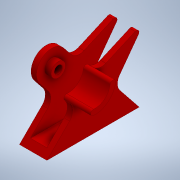
# Autodesk Inventor part: WeaponMountV1
Saved by Autodesk Inventor 2020 (Build 240168000, 168)
## iProperties
Created: 2024-02-06
Part Number: WeaponMountV1
Material: PETG
Document SubType Name: Modeling
Designer: smz3rm
Density: 1 g/cm^3
Appearance: Generic
Mass: 35.5696 g
Surface Area: 166.474 cm^2
Volume: 35.5696 cm^3
Author: smz3rm
Autodesk Inventor part; units mm, degrees
ref_plane "YZ Plane" through (0, 0, 0) normal (1, 0, 0) x (0, 1, 0)
ref_plane "XZ Plane" through (0, 0, 0) normal (0, 1, 0) x (-1, 0, 0)
ref_plane "XY Plane" through (0, 0, 0) normal (0, 0, 1) x (1, 0, 0)
sketch "Sketch1" plane through (0, 0, 0) normal (1, 0, 0) x (0, 1, 0)
  line L0 (0, 0) -> (27, -27)
  line L1 (27, -27) -> (0, -27)
  line L2 (0, -27) -> (0, 0)
  circle A0 centre (52.45, -24.45) radius 2.5
  line L3 (61.129583, -35.307018) -> (0, -84.176728)
  line L4 (0, -84.176728) -> (0, -27)
  circle A1 centre (52.45, -24.45) radius 13.9
  line L5 (27, -27) -> (43.770417, -13.592982)
  point P0 (0, -27)
  dimension "d0" = 45
  dimension "d1" = 27
  dimension "d2" = 5
  dimension "d10" = 52.45
  dimension "d12" = 24.45
  dimension "d34" = 27.8
  dimension "d38" = 51.3596
  constraints: 12 end point, 2 centre point, 2 coincident, 2 point on circle, 2 tangent, 1 collinear, 1 horizontal, 1 parallel, 1 perpendicular, 1 vertical
  measures "d0" angle of L2 L0
  measures "d1" distance of L0.end L1.end
  measures "d2" diameter of A0
  measures "d10" distance from line of L2 A0.centre
  measures "d12" vertical distance of A0.centre L0.start
  measures "d34" diameter of A1
  measures "d38" angle of L4 L3
extrude "Extrusion1" add sketch "Sketch1" along normal blind 5
sketch "Sketch2" plane through (5, 0, 0) normal (1, 0, 0) x (0, 0, -1)
  line L0 (27, 27) -> (0, 0)
  line L1 (5, 5) -> (91.557569, 5)
  arc A0 (35.307018, 61.129583) -> (13.592982, 43.770417) centre (24.45, 52.45) ccw
  line L2 (0, 0) -> (84.176728, 0)
  line L3 (84.176728, 0) -> (35.307018, 61.129583)
  line L4 (13.592982, 43.770417) -> (27, 27)
  point P0 (80.179505, 5)
  constraints: 2 end point, 1 horizontal, 1 point on line
extrude "Extrusion2" add sketch "Sketch2" along normal blind 15 contours L1 L3 L2 L0
sketch "Sketch3" plane through (5, 0, 0) normal (1, 0, 0) x (0, 0, -1)
  circle A0 centre (24.45, 52.45) radius 2.5
  circle A1 centre (24.45, 52.45) radius 3.65
  circle A2 centre (24.45, 52.45) radius 6.5
  arc A3 (35.307018, 61.129583) -> (13.592982, 43.770417) centre (24.45, 52.45) ccw
  line L0 (5, 5) -> (80.179505, 5)
  line L1 (80.179505, 5) -> (35.307018, 61.129583)
  line L2 (13.592982, 43.770417) -> (27, 27)
  line L3 (27, 27) -> (5, 5)
  point P0 (0, 0)
  dimension "d14" = 7.3
  dimension "d15" = 13
  constraints: 2 centre point, 2 coincident
  measures "d14" diameter of A1
  measures "d15" diameter of A2
extrude "Extrusion3" add sketch "Sketch3" along normal blind 6 contours A2
ref_plane "Work Plane1" through (12.5, 0, 0) normal (1, 0, 0) x (0, 0, -1)
mirror "Mirror1" about plane through (12.5, 0, 0) normal (1, 0, 0) of "Extrusion1"
sketch "Sketch4" plane through (25, 46.692431, -5.55) normal (1, 0, 0) x (0, 0, -1)
  circle A0 centre (18.9, 5.757569) radius 2.5
  circle A1 centre (18.9, 5.757569) radius 13.9
  line L0 (21.45, -19.692431) -> (-5.55, -46.692431)
  arc A2 (29.757018, 14.437152) -> (8.042982, -2.922015) centre (18.9, 5.757569) ccw
  line L1 (-5.55, -46.692431) -> (78.626728, -46.692431)
  line L2 (78.626728, -46.692431) -> (29.757018, 14.437152)
  line L3 (8.042982, -2.922015) -> (21.45, -19.692431)
  dimension "d19" = 27.8
  constraints: 1 centre point, 1 coincident
  measures "d19" diameter of A1
extrude "Extrusion4" cut sketch "Sketch4" against normal up to surface (5 mm away) contours A0 | A1
sketch "Sketch5" plane through (25, 0, 0) normal (1, 0, 0) x (0, 0, -1)
  circle A0 centre (24.45, 52.45) radius 6.5
  arc A1 (22.90761, 36.122691) -> (40.716243, 50.359705) centre (24.45, 52.45) ccw construction
  arc A2 (22.672489, 33.633771) -> (43.195853, 50.041062) centre (24.45, 52.45) ccw
  arc A3 (23.14273, 38.61161) -> (38.236633, 50.678347) centre (24.45, 52.45) ccw
  arc A4 (23.14273, 38.61161) -> (22.672489, 33.633771) centre (22.90761, 36.122691) ccw
  arc A5 (43.195853, 50.041062) -> (38.236633, 50.678347) centre (40.716243, 50.359705) ccw
  line L0 (84.176728, 0) -> (35.307018, 61.129583)
  arc A6 (13.592982, 43.770417) -> (35.307018, 61.129583) centre (24.45, 52.45) ccw
  line L1 (13.592982, 43.770417) -> (27, 27)
  point P0 (0, 0)
  point P1 (96.557569, 0)
  point P2 (36.312855, 54.630693)
  point P3 (42.61545, 53.942118)
  point P4 (96.557569, 0)
  point P5 (42.61545, 53.942118)
  point P6 (42.668944, 51.920781)
  point P7 (20.954909, 34.561614)
  dimension "d22" = 13.9
  dimension "d23" = 5
  constraints: 10 point on circle, 5 centre point, 5 tangent, 1 coincident, 2 other
  measures "d22" radius of A3
  measures "d23" radial gap between concentric circles of A3 A2
extrude "Extrusion5" cut sketch "Sketch5" against normal up to surface (5 mm away) contours L1 A6 A4 | A5 A6 L0
extrude "Extrusion6" add sketch "Sketch5" along normal blind 19.5 contours A4 A3 A5 A2
sketch "Sketch6" plane through (25, 0, 0) normal (1, 0, 0) x (0, 0, -1)
  line L0 (27, 27) -> (0, 0)
  line L1 (80.179505, 5) -> (42.668944, 51.920781)
  circle A0 centre (81.589292, 59.287621) radius 2.5
  line L2 (46.779285, 46.779285) -> (80.586804, 61.577821)
  line L3 (61.723669, 28.085825) -> (83.602572, 57.805493)
  line L4 (27, 27) -> (46.779285, 46.779285)
  line L5 (27, 27) -> (0, 0)
  point P0 (5, 5)
  point P1 (42.668944, 51.920781)
  point P2 (96.557569, 0)
  point P3 (42.668944, 51.920781)
  dimension "d31" = 5
  dimension "d32" = 30
  dimension "d33" = 35
  constraints: 6 end point, 2 point on circle, 2 tangent, 1 centre point, 1 collinear, 1 equal length, 3 other
  measures "d31" diameter of A0
  measures "d32" angle of L2 L3
extrude "Extrusion7" add sketch "Sketch6" against normal up to surface (5 mm away)
mirror "Mirror2" about plane through (12.5, 0, 0) normal (1, 0, 0) of "Extrusion7"
fillet "Fillet1" radius 10 6 edges at (22.5, 46.7793, -46.7793) (2.5, 46.7793, -46.7793) (22.5, 28.0858, -61.7237) (2.5, 28.0858, -61.7237) (2.5, 27, -27) (22.5, 27, -27)
equation "\"d0\" = FrontAngle"
equation "\"d1\" = Height - BaseThickness"
equation "\"d10\" = WeaponHeight + WeaponMountThickness"
equation "\"d12\" = 0.5 * WeaponDia - WeaponBite"
equation "\"d34\" = WeaponMotorDia"
equation "\"d5\" = WeaponMountThickness"
equation "\"d8\" = WeaponOpeningWidth"
equation "\"d19\" = WeaponMotorDia"
equation "\"d22\" = 0.5 * WeaponMotorDia"
equation "\"d23\" = WeaponMountThickness"
equation "\"d24\" = WeaponMountThickness"
equation "\"d26\" = -0.5 * WeaponOpeningWidth + WeaponCenterToMotorBack - WeaponMountThickness"
equation "\"WeaponDia\" = 88.9"
equation "\"d18\" = 0.5 * WeaponOpeningWidth"
equation "\"WeaponMotorDia\" = 27.8"
equation "\"FrontAngle\" = 45deg"
equation "\"Height\" = 30"
equation "\"BaseThickness\" = 3"
equation "\"WeaponHeight\" = 47.45"
equation "\"WeaponMountThickness\" = 5"
equation "\"WeaponBite\" = 20"
equation "\"WeaponOpeningWidth\" = 15"
equation "\"WeaponCenterToMotorBack\" = 32"
body "Solid1"
